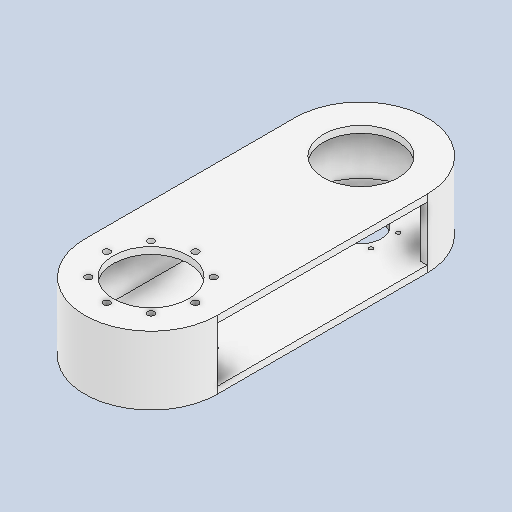
# Autodesk Inventor part: joint1_frame
Saved by Autodesk Inventor 2025.3 (Build 293356030, 356C)
## iProperties
Created: 2025-09-07
Part Number: joint1_frame
Material: PLA+ filament
Document SubType Name: Modeling
Designer: MSI
Mass: 333.016 g
Surface Area: 1149.86 cm^2
Volume: 270.745 cm^3
Density: 1.23 g/cm^3
Appearance: 일반
Author: MSI
Autodesk Inventor part; units mm, degrees
ref_plane "YZ Plane" through (0, 0, 0) normal (1, 0, 0) x (0, 1, 0)
ref_plane "XZ Plane" through (0, 0, 0) normal (0, 1, 0) x (-1, 0, 0)
ref_plane "XY Plane" through (0, 0, 0) normal (0, 0, 1) x (1, 0, 0)
sketch "스케치1" plane through (0, 0, 0) normal (0, 1, 0) x (-1, 0, 0)
  line L0 (0, 0) -> (0, 153.831) construction
  line L1 (48.5, 0) -> (48.5, 153.831)
  line L2 (-48.5, 153.831) -> (-48.5, 0)
  arc A0 (-48.5, 0) -> (48.5, 0) centre (0, 0) ccw
  arc A1 (48.5, 153.831) -> (-48.5, 153.831) centre (0, 153.831) ccw
  point P0 (0, 76.9155)
  dimension "d0" = 48.5
  dimension "d1" = 153.831
  constraints: 8 end point, 4 point on circle, 4 tangent, 2 centre point, 1 midpoint, 1 parallel, 1 vertical
  measures "d0" radius of A0
  measures "d1" distance of L1.start L1.end
extrude "돌출1" add sketch "스케치1" along normal blind 50
shell "쉘1" thickness 5 removed faces 0
sketch "스케치2" plane through (48.5, 0, 153.831) normal (1, 0, 0) x (0, 0, -1)
  line L0 (0, 45) -> (153.831, 45) projected
  line L1 (197.331, 5) -> (153.831, 5) projected
  line L2 (0, 45) -> (153.831, 45)
  line L3 (153.831, 45) -> (153.831, 5)
  line L4 (153.831, 5) -> (0, 5)
  line L5 (0, 5) -> (0, 45)
  point P0 (153.831, 0)
  constraints: 8 end point, 2 parallel, 1 horizontal, 1 perpendicular
extrude "돌출2" cut sketch "스케치2" against normal blind 5
sketch "스케치3" plane through (0, 50, 0) normal (0, 1, 0) x (1, 0, 0)
  arc A0 (-43.5, -153.831) -> (43.5, -153.831) centre (0, -153.831) ccw projected
  circle A1 centre (0, -153.831) radius 27.5
  point P0 (0, 0)
  dimension "d10" = 55
  constraints: 1 centre point, 1 coincident
  measures "d10" diameter of A1
extrude "돌출3" cut sketch "스케치3" against normal through all
sketch "스케치4" plane through (0, 50, 0) normal (0, 1, 0) x (1, 0, 0)
  circle A0 centre (0, -153.831) radius 27.5 projected
  line L0 (0, -153.831) -> (32.5, -153.831) construction
  point P0 (0, 0)
  dimension "d13" = 32.5
  constraints: 2 end point, 1 coincident, 1 horizontal
  measures "d13" distance of L0.start L0.end
hole "구멍1" at (32.5, 50, 153.831) direction (0, -1, 0) diameter 5 end through all
pattern_circular "원형 패턴1" count 8 over 360 about axis through (0, 50, 153.831) along (0, -1, 0) of "구멍1"
sketch "스케치5" plane through (0, 50, 0) normal (0, 1, 0) x (1, 0, 0)
  arc A0 (48.5, 0) -> (-48.5, 0) centre (0, 0) ccw projected
  constraints: 1 coincident
hole "구멍2" at (0, 50, 0) direction (0, -1, 0) diameter 30 end through all counterbore diameter 55 counterbore depth 5
sketch "스케치6" plane through (0, 0, 0) normal (0, -1, 0) x (1, 0, 0)
  line L0 (0, 0) -> (0, 20) construction
  dimension "d31" = 20
  constraints: 2 end point, 1 vertical
  measures "d31" distance of L0.start L0.end
hole "구멍3" at (0, 0, 20) direction (0, 1, 0) diameter 2.9 depth 5 clearance for "Flat Head Machine Screw" size "M2.5" standard "Ansi Metric M Profile"
pattern_circular "원형 패턴2" count 6 over 360 about axis through (0, -223.5419, 0) along (0, 1, 0) of "구멍3"
